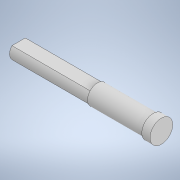
# Autodesk Inventor part: draaiarm voorwielen
Saved by Autodesk Inventor 2022 (Build 260153000, 153)
## iProperties
Created: 2021-12-08
Part Number: draaiarm voorwielen
Material: Generic
Document SubType Name: Modeling
Designer: keemi
Density: 1 g/cm^3
Appearance: Default
Author: keemi
Autodesk Inventor part; units mm, degrees
ref_plane "YZ Plane" through (0, 0, 0) normal (1, 0, 0) x (0, 1, 0)
ref_plane "XZ Plane" through (0, 0, 0) normal (0, 1, 0) x (-1, 0, 0)
ref_plane "XY Plane" through (0, 0, 0) normal (0, 0, 1) x (1, 0, 0)
sketch "Sketch1" plane through (0, 0, 0) normal (1, 0, 0) x (0, 1, 0)
  circle A0 centre (0, 0) radius 3
  dimension "d0" = 6
  constraints: 1 centre point, 1 coincident
  measures "d0" diameter of A0
extrude "Extrusion1" add sketch "Sketch1" along normal blind 17
sketch "Sketch2" plane through (17, 0, 0) normal (1, 0, 0) x (0, 0, -1)
  circle A0 centre (0, 0) radius 3.45
  dimension "d3" = 6.9
  constraints: 1 centre point, 1 coincident
  measures "d3" diameter of A0
extrude "Extrusion2" add sketch "Sketch2" along normal blind 2.5
sketch "Sketch3" plane through (0, 0, 0) normal (-1, 0, 0) x (0, 0, 1)
  circle A0 centre (0, 0) radius 2.75
  dimension "d6" = 5.5
  constraints: 1 centre point, 1 coincident
  measures "d6" diameter of A0
extrude "Extrusion3" add sketch "Sketch3" along normal blind 24
sketch "Sketch4" plane through (-24, 0, 0) normal (-1, 0, 0) x (0, 0, 1)
  line L0 (0, 0) -> (0, -1.85)
  line L1 (0, 0) -> (0, 1.85)
  line L2 (0, -1.85) -> (-3.7501, -1.85)
  line L3 (-3.7501, -1.85) -> (3.8768, -1.85)
  line L4 (3.8768, -1.85) -> (3.8768, 1.85)
  line L5 (3.8768, 1.85) -> (-3.7501, 1.85)
  line L6 (-3.7501, 1.85) -> (-3.7501, -1.85)
  line L7 (-7.0983, -8.0342) -> (8.0665, -8.0342)
  line L8 (8.0665, -8.0342) -> (8.0665, 8.0154)
  line L9 (8.0665, 8.0154) -> (-7.0983, 8.0154)
  line L10 (-7.0983, 8.0154) -> (-7.0983, -8.0342)
  dimension "d9" = 1.85
  dimension "d10" = 1.85
  constraints: 22 end point, 4 parallel, 3 horizontal, 2 perpendicular, 2 vertical
  measures "d9" distance of L0.start L0.end
  measures "d10" distance of L0.start L1.end
extrude "Extrusion4" cut sketch "Sketch4" against normal blind 24
body "Solid1"
